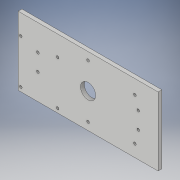
# Autodesk Inventor part: Деталь1
Saved by Autodesk Inventor 2019.2 (Build 232265000, 265)
## iProperties
Created: 2023-02-24
Part Number: Деталь1
Material: Типовые
Document SubType Name: Modeling
Designer: Преподаватель
Density: 1 g/cm^3
Appearance: По умолчанию
Author: Преподаватель
Autodesk Inventor part; units mm, degrees
ref_plane "YZ Plane" through (0, 0, 0) normal (1, 0, 0) x (0, 1, 0)
ref_plane "XZ Plane" through (0, 0, 0) normal (0, 1, 0) x (-1, 0, 0)
ref_plane "XY Plane" through (0, 0, 0) normal (0, 0, 1) x (1, 0, 0)
sketch "Эскиз1" plane through (0, 0, 0) normal (0, 0, 1) x (1, 0, 0)
  line L0 (0, 0) -> (-184, 0)
  line L1 (-184, 0) -> (-184, 90)
  line L2 (-184, 90) -> (0, 90)
  line L3 (0, 90) -> (0, 0)
  dimension "d0" = 184
  dimension "d1" = 90
  constraints: 8 end point, 3 perpendicular, 1 horizontal
  measures "d0" distance of L0.start L0.end
  measures "d1" distance of L0.end L1.end
extrude "Выдавливание1" add sketch "Эскиз1" along normal blind 5
sketch "Эскиз2" plane through (0, 0, 5) normal (0, 0, 1) x (1, 0, 0)
  line L0 (0, 90) -> (-184, 90) projected
  line L1 (-26, 45) -> (-26, 56)
  line L2 (-26, 56) -> (-158, 56)
  line L3 (-158, 56) -> (-158, 34)
  line L4 (-158, 34) -> (-26, 34)
  line L5 (-26, 34) -> (-26, 56)
  circle A0 centre (-158, 56) radius 1.75
  circle A1 centre (-26, 56) radius 1.75
  circle A2 centre (-26, 34) radius 1.75
  circle A3 centre (-158, 34) radius 1.75
  point P0 (0, 0)
  dimension "d43" = 11
  dimension "d44" = 132
  dimension "d45" = 22
  dimension "d46" = 3.5
  dimension "d47" = 3.5
  dimension "d48" = 3.5
  dimension "d49" = 3.5
  constraints: 10 end point, 4 centre point, 4 coincident, 2 parallel, 1 horizontal, 1 perpendicular
  measures "d43" distance of L1.start L1.end
  measures "d44" distance of L4.end L3.end
  measures "d45" distance of L3.end L2.end
  measures "d46" diameter of A0
  measures "d47" diameter of A1
  measures "d48" diameter of A2
  measures "d49" diameter of A3
extrude "Выдавливание2" cut sketch "Эскиз2" against normal blind 5 contours A1 L2 L1 | L1 L2 A1 | A2 L4 L5 | L5 L4 A2 | A0 L3 L2 | L2 L3 A0 | A3 L3 L4 | L4 L3 A3
sketch "Эскиз8" plane through (0, 0, 5) normal (0, 0, 1) x (1, 0, 0)
  line L0 (-184, 0) -> (-184, 90) projected
  line L1 (-184, 0) -> (-92, 0)
  line L2 (0, 0) -> (-184, 0) projected
  line L3 (-92, 0) -> (-92, 10)
  line L4 (-92, 10) -> (-92, 80)
  circle A0 centre (-92, 80) radius 1.75
  circle A1 centre (-92, 10) radius 1.75
  dimension "d52" = 92
  dimension "d53" = 10
  dimension "d54" = 70
  dimension "d55" = 3.5
  dimension "d56" = 3.5
  constraints: 6 end point, 2 centre point, 2 coincident, 1 midpoint, 1 perpendicular, 1 point on line
  measures "d52" distance of L0.start L1.end
  measures "d53" distance of L1.end L3.end
  measures "d54" distance of L3.end L4.end
  measures "d55" diameter of A0
  measures "d56" diameter of A1
extrude "Выдавливание3" cut sketch "Эскиз8" against normal blind 5
sketch "Эскиз9" plane through (0, 0, 5) normal (0, 0, 1) x (1, 0, 0)
  line L0 (0, 90) -> (0, 85)
  line L1 (0, 90) -> (0, 0) projected
  line L2 (-60, 85) -> (-60, 5)
  line L3 (-60, 5) -> (0, 5)
  line L4 (0, 5) -> (0, 85)
  line L5 (-184, 90) -> (-184, 87.5)
  line L6 (-184, 0) -> (-184, 90) projected
  line L7 (-184, 0) -> (-184, 2.5)
  line L8 (-129, 87.5) -> (-129, 2.5)
  line L9 (-129, 2.5) -> (-184, 2.5)
  line L10 (-184, 2.5) -> (-184, 87.5)
  line L11 (-60, 77) -> (-129, 77)
  line L12 (-129, 87.5) -> (-129, 63.5)
  line L13 (-129, 63.5) -> (-132, 63.5)
  circle A0 centre (-132, 63.5) radius 1.75
  circle A1 centre (-180.5, 63.5) radius 1.75
  circle A2 centre (-132, 5.5) radius 1.75
  circle A3 centre (-180.5, 5.5) radius 1.75
  line L14 (-180.5, 63.5) -> (-180.5, 5.5)
  line L15 (-180.5, 5.5) -> (-132, 5.5)
  line L16 (-132, 5.5) -> (-132, 63.5)
  line L17 (-60, 5) -> (-30.5, 5)
  line L18 (-30.5, 5) -> (-30.5, 16)
  circle A4 centre (-30.5, 16) radius 1.75
  line L19 (-30.5, 16) -> (-30.5, 71.5)
  circle A5 centre (-30.5, 71.5) radius 1.75
  dimension "d61" = 5
  dimension "d62" = 60
  dimension "d63" = 80
  dimension "d64" = 2.5
  dimension "d65" = 2.5
  dimension "d66" = 55
  dimension "d67" = 85
  dimension "d69" = 69
  dimension "d70" = 24
  dimension "d71" = 3
  dimension "d72" = 3.5
  dimension "d75" = 3.5
  dimension "d76" = 3.5
  dimension "d77" = 3.5
  dimension "d78" = 58
  dimension "d79" = 48.5
  dimension "d80" = 29.5
  dimension "d81" = 11
  dimension "d82" = 3.5
  dimension "d83" = 55.5
  dimension "d84" = 3.5
  constraints: 36 end point, 7 point on line, 6 centre point, 3 coincident, 3 parallel, 3 perpendicular, 1 vertical
  measures "d61" distance of L0.start L0.end
  measures "d62" distance of L3.end L2.end
  measures "d63" distance of L2.end L2.start
  measures "d64" distance of L5.start L5.end
  measures "d65" distance of L6.start L7.end
  measures "d66" distance of L8.end L9.end
  measures "d67" distance of L8.start L8.end
  measures "d69" distance of L11.start L11.end
  measures "d70" distance of L8.start L12.end
  measures "d71" distance of L12.end L13.end
  measures "d72" diameter of A0
  measures "d75" diameter of A1
  measures "d76" diameter of A2
  measures "d77" diameter of A3
  measures "d78" distance of L14.start L14.end
  measures "d79" distance of L16.end L14.start
  measures "d80" distance of L2.end L17.end
  measures "d81" distance of L17.end L18.end
  measures "d82" diameter of A4
  measures "d83" distance of L19.start L19.end
  measures "d84" diameter of A5
extrude "Выдавливание4" cut sketch "Эскиз9" against normal blind 5
sketch "Эскиз10" plane through (0, 0, 5) normal (0, 0, 1) x (1, 0, 0)
  line L0 (0, 0) -> (-184, 0) projected
  circle A0 centre (-92, 45) radius 10
  dimension "d89" = 20
  constraints: 1 centre point
  measures "d89" diameter of A0
extrude "Выдавливание5" cut sketch "Эскиз10" against normal blind 5
